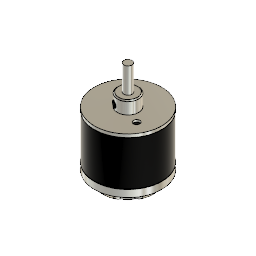
Propeller Shroud 3 (Not finished) v12 (Autodesk Fusion 360 archive; units mm, degrees)
design "M100 motor"
Autodesk Fusion 360 part; units mm, degrees
note: some values were not read from the file. Chosen so that the rebuilt part matches the saved one: which face or edge a step refers to; where a thread starts. Set by a fixed rule: which sketch regions a step uses.
sketch "Sketch1" plane through (0, 0, 0) normal (0, 0, 1) x (1, 0, 0)
  circle A0 centre (0, 0) radius 16
  dimension "d103_1" = 32
  measures "d103_1" diameter of A0
extrude "Extrude1" add sketch "Sketch1" against normal blind 22.7 makes body 1
extrude "Extrude2" add 1 faces at (3.3126, -0.5422, -22.7) along direction (0, 0, -1) blind 7.3 separate body on bodies 1 makes body 2
chamfer "Chamfer1" distance 4 angle 45 1 edges at (-14.9172, 5.7858, -30) on bodies 2
extrude "Extrude3" cut 1 faces at (3.3126, -0.5422, 0) along direction (0, 0, -1) blind 1.5 on bodies 1 bodies 1
extrude "Extrude4" add 1 faces at (3.3126, -0.5422, -1.5) along direction (0, 0, 1) blind 1.5 separate body on bodies 1 makes body 3
sketch "Sketch2" plane through (0, 0, -30) normal (0, 0, -1) x (1, 0, 0)
  circle A0 centre (0, 0) radius 12
  circle A1 centre (0, 0) radius 1.975
  dimension "d113_1" = 3.95
  measures "d113_1" diameter of A1
extrude "Extrude5" cut sketch "Sketch2" against normal up to surface (30 mm away) contours A1 bodies 1 2 3
sketch "Sketch3" plane through (0, 0, 0) normal (0, 0, 1) x (1, 0, 0)
  circle A0 centre (0, 0) radius 5
  dimension "d116_1" = 10
  measures "d116_1" diameter of A0
extrude "Extrude6" add sketch "Sketch3" along normal blind 6 bodies 3
chamfer "Chamfer2" distance 0.5 angle 45 1 edges at (-4.6616, -1.8081, 6) on bodies 3
sketch "Sketch4" plane through (0, 0, 6) normal (0, 0, 1) x (-1, 0, 0)
  circle A0 centre (0, 0) radius 4.5
  circle A1 centre (0, 0) radius 1.975
extrude "Extrude7" add sketch "Sketch4" along normal blind 12 contours A1 bodies 3
sketch "Sketch5" plane through (0, 0, -30) normal (0, 0, -1) x (1, 0, 0)
  circle A0 centre (0, 0) radius 1.975
  circle A1 centre (0, 0) radius 12
  circle A2 centre (0, 0) radius 5
  dimension "d122_1" = 10
  measures "d122_1" diameter of A2
extrude "Extrude8" add sketch "Sketch5" along normal blind 5 separate body contours A2 makes body 4
extrude "Extrude9" add 1 faces at (0.6904, -0.271, 0) along direction (0, 0, -1) blind 35.7 on bodies 3 bodies 3 4
chamfer "Chamfer3" distance 0.25 angle 45 1 edges at (-4.6616, 1.8081, -35) on bodies 3 4
chamfer "Chamfer4" distance 0.25 angle 45 1 edges at (-4.6616, 1.8081, -30) on bodies 3 4
sketch "Sketch6" plane through (0, 0, 0) normal (0, 1, 0) x (1, 0, 0)
  circle A0 centre (0, -2) radius 1.5
  dimension "d129_1" = 3
  measures "d129_1" diameter of A0
extrude "Extrude10" cut sketch "Sketch6" along normal blind 6 bodies 3
extrude "Extrude11" add 1 faces at (0.3117, 0, 2.3909) along direction (0, 1, 0) blind 5 and the other way blind -3 separate body on bodies 3 makes body 5
thread "Thread1" "ISO Metric profile 3.0 M3x0.5 6g" major diameter 2.927 minor diameter 2.3555 pitch 0.5 angle 60 modelled right hand crest width 0.0625 on face at (1.4925, 4.3333, 2.1494) crest through (1.4635, 2.9688, 2) on bodies 5
sketch "Sketch7" plane through (0, 5, 0) normal (0, 1, 0) x (-1, 0, 0)
  line L0 (-0.433, 2.75) -> (-0.866, 2)
  line L1 (-0.866, 2) -> (-0.433, 1.25)
  line L2 (-0.433, 1.25) -> (0.433, 1.25)
  line L3 (0.433, 1.25) -> (0.866, 2)
  line L4 (0.866, 2) -> (0.433, 2.75)
  line L5 (0.433, 2.75) -> (-0.433, 2.75)
  spline S0 degree 3 poles (-1.0349, 0.9651) (-0.8913, 0.8463) (-0.7262, 0.7561) (-0.377, 0.6473) (-0.1971, 0.6273) (0.1534, 0.6581) (0.3207, 0.706) (0.6209, 0.8612) (0.752, 0.9647) (0.9302, 1.1745) (0.9899, 1.2673) (1.0813, 1.4637) (1.1132, 1.5659) (1.1309, 1.6711) knots 0 0 0 0 0.055923 0.055923 0.109803 0.109803 0.161639 0.161639 0.211432 0.211432 0.244511 0.244511 0.276632 0.276632 0.276632 0.276632
  arc A0 (1.1309, 1.6711) -> (0.5671, 3.0322) centre (0, 2) ccw
  spline S1 degree 3 poles (0.5671, 3.0322) (0.4403, 3.1225) (0.2968, 3.1867) (-0.0133, 3.2591) (-0.1774, 3.2643) (-0.5055, 3.2115) (-0.6659, 3.1515) (-0.9612, 2.9709) (-1.092, 2.8498) (-1.271, 2.6056) (-1.3314, 2.4942) (-1.4221, 2.2554) (-1.4514, 2.1288) (-1.4635, 2) knots 0 0 0 0 0.046698 0.046698 0.095434 0.095434 0.146206 0.146206 0.199015 0.199015 0.236706 0.236706 0.275362 0.275362 0.275362 0.275362
  arc A1 (-1.4635, 2) -> (-1.0349, 0.9651) centre (0, 2) ccw
  dimension "d136_1" = 0.75
  measures "d136_1" distance of L5
extrude "Extrude12" cut sketch "Sketch7" against normal blind 1 contours L0 L1 L2 L3 L4 L5 bodies 5
sketch "Sketch8" plane through (0, 0, 0) normal (0, 1, 0) x (1, 0, 0)
  circle A0 centre (0, 32.5) radius 1.5
  dimension "d139_1" = 3
  measures "d139_1" diameter of A0
extrude "Extrude13" cut sketch "Sketch8" along normal blind 5.5 and the other way blind -2 bodies 3
extrude "Extrude14" add 1 faces at (-0.3239, 2, -32.9442) along direction (0, 1, 0) blind 3 separate body on bodies 3 makes body 6
sketch "Sketch9" plane through (0, 5, 0) normal (0, 1, 0) x (-1, 0, 0)
  circle A0 centre (0, -32.5) radius 1.5
  line L0 (-0.433, -31.75) -> (-0.866, -32.5)
  line L1 (-0.866, -32.5) -> (-0.433, -33.25)
  line L2 (-0.433, -33.25) -> (0.433, -33.25)
  line L3 (0.433, -33.25) -> (0.866, -32.5)
  line L4 (0.866, -32.5) -> (0.433, -31.75)
  line L5 (0.433, -31.75) -> (-0.433, -31.75)
  dimension "d146_1" = 0.75
extrude "Extrude15" cut sketch "Sketch9" against normal blind 1 contours L0 L1 L2 L3 L4 L5 bodies 6
thread "Thread2" "ISO Metric profile 3.0 M3x0.5 6g" major diameter 2.927 minor diameter 2.3555 pitch 0.5 angle 60 modelled right hand crest width 0.0625 on face at (-1.3173, 4, -33.2174) crest through (1.4635, 1.9688, -32.5) on bodies 6
sketch "Sketch10" plane through (0, 0, 0) normal (0, 0, 1) x (-1, 0, 0)
  circle A0 centre (0, 0) radius 5
  circle A1 centre (0, 0) radius 16
  circle A2 centre (0, 0) radius 9.55 construction
  circle A3 centre (-9.55, 0) radius 1.5
  line L0 (0, 0) -> (0, 6.7707) construction
  circle A4 centre (9.55, 0) radius 1.5
  dimension "d149_1" = 19.1
  dimension "d150_1" = 3
  measures "d149_1" diameter of A2
  measures "d150_1" diameter of A3
extrude "Extrude16" cut sketch "Sketch10" against normal blind 1 contours A3 | A4 bodies 3
thread "Thread3" [suppressed]
sketch "Sketch11" plane through (0, 0, -30) normal (0, 0, -1) x (1, 0, 0)
  circle A0 centre (0, 0) radius 1.975
  circle A1 centre (0, 0) radius 12
  circle A2 centre (0, 0) radius 9.5 construction
  circle A3 centre (9.5, 0) radius 1.5
  line L0 (0, -6.5) -> (0, 3.5) construction
  circle A4 centre (-9.5, 0) radius 1.5
  line L1 (0, 0) -> (1.975, 0) construction
  circle A5 centre (0, 0) radius 8 construction
  circle A6 centre (0, -8) radius 1.5
  circle A7 centre (0, 8) radius 1.5
  circle A8 centre (0, 0) radius 16
  line L2 (0, 0) -> (11.3137, 11.3137) construction
  line L3 (0, 0) -> (16, 0) construction
  line L4 (4.4495, 11.6824) -> (11.1722, 4.2794)
  line L5 (11.1722, 4.2794) -> (14.8737, 7.6408)
  line L6 (14.8737, 7.6408) -> (8.151, 15.0438)
  line L7 (8.151, 15.0438) -> (4.4495, 11.6824)
  line L8 (4.4495, 11.6824) -> (14.8737, 7.6408) construction
  line L9 (11.1722, 4.2794) -> (8.151, 15.0438) construction
  dimension "d153_1" = 19
  dimension "d154_1" = 3
  dimension "d159_1" = 19
  dimension "d160_1" = 16
  dimension "d161_1" = 3
  dimension "d164_1" = 45
  dimension "d165_1" = 10
  dimension "d166_1" = 5
  measures "d153_1" diameter of A2
  measures "d154_1" diameter of A3
  measures "d159_1" diameter of A2
  measures "d160_1" diameter of A5
  measures "d161_1" diameter of A6
  measures "d164_1" angle of L2 L3
extrude "Extrude19" cut sketch "Sketch11" against normal blind 4 contours A1 L4 L5 | A1 A8 L4 L5 L7 | A8 L5 L6 L7 picked at (7.7523, 8.3123) picked at (12.6834, 7.3216) bodies 2
extrude "Extrude18" cut sketch "Sketch11" against normal blind 2 contours A3 | A4 | A6 | A7 bodies 2
thread "Thread4" [suppressed]
fillet "Fillet1" radius 2.5 2 edges at (4.4495, -11.6824, -27.7495) (11.1722, -4.2794, -28) on bodies 2
copy_body "CutPasteBodies1" bodies 2 removing the originals makes body 7 in component "Static parts"
copy_body "CutPasteBodies1'" bodies 1 removing the originals makes body 8 in component "Moving parts"
copy_body "CutPasteBodies2" bodies 3 removing the originals makes body 9 in component "Moving parts"
copy_body "CutPasteBodies3" bodies 5 removing the originals makes body 10 in component "Moving parts"
copy_body "CutPasteBodies4" bodies 6 removing the originals makes body 11 in component "Moving parts"
component "Static parts" placed x (1, 0, 0) y (0, 1, 0) z (0, 0, 1) at (0, 0, 0)
component "Moving parts" placed x (-0.888292, 0.459279, 0) y (-0.459279, -0.888292, 0) z (0, 0, 1) at (0, 0, 0.099)
